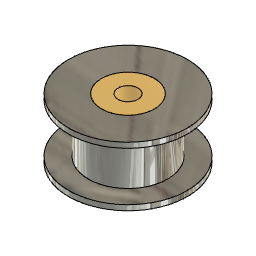
ZSync_Belt_Tensioner_-_Alt_3_v16 (Autodesk Fusion 360 archive; units mm, degrees)
design "Idler Pulley"
Autodesk Fusion 360 part; units mm, degrees
sketch "Sketch1" plane through (0, 0, 0) normal (0, 0, 1) x (1, 0, 0)
  circle A0 centre (0, 0) radius 1.5
  circle A1 centre (0, 0) radius 4
  circle A2 centre (0, 0) radius 6
  circle A3 centre (0, 0) radius 9
  dimension "d1" = 3
  dimension "d2" = 8
  dimension "d3" = 12
  dimension "d4" = 18
  constraint coincident A0.centre A1.centre
  constraint concentric A0 A1
  constraint concentric A1 A2
  constraint concentric A0 A3
  measures "d1" diameter of A0
  measures "d2" diameter of A1
  measures "d3" diameter of A2
  measures "d4" diameter of A3
extrude "Extrude1" add sketch "Sketch1" along normal blind 9 contours A1 makes body 1
extrude "Extrude2" add sketch "Sketch1" along normal blind 9 separate body contours A2 makes body 2
extrude "Extrude3" add sketch "Sketch1" along normal blind 0.8 contours A3 bodies 2
extrude "Extrude4" add sketch "Sketch1" against normal blind 0.8 from surface at 9 contours A3 bodies 2
